Autodesk Fusion 360 part; units mm, degrees
(part 2 of 2)
  measures "d325" diameter of A232
  measures "d326" diameter of A227
  measures "d327" diameter of A198
  measures "d328" diameter of A280
  measures "d329" diameter of A253
  measures "d330" diameter of A200
  measures "d331" diameter of A269
  measures "d332" diameter of A224
  measures "d333" diameter of A233
  measures "d334" diameter of A214
  measures "d335" diameter of A265
  measures "d336" diameter of A279
  measures "d337" diameter of A204
  measures "d338" diameter of A298
  measures "d339" diameter of A210
  measures "d340" diameter of A157
  measures "d341" diameter of A205
  measures "d342" diameter of A155
  measures "d343" diameter of A225
  measures "d344" diameter of A202
  measures "d345" diameter of A241
  measures "d346" diameter of A270
  measures "d347" diameter of A262
  measures "d348" diameter of A208
  measures "d349" diameter of A301
  measures "d350" diameter of A240
  measures "d351" diameter of A197
  measures "d352" diameter of A231
  measures "d353" diameter of A264
  measures "d354" diameter of A267
  measures "d355" diameter of A213
  measures "d356" diameter of A297
  measures "d357" diameter of A164
  measures "d358" diameter of A178
  measures "d359" diameter of A194
  measures "d360" diameter of A296
  measures "d361" diameter of A180
  measures "d362" diameter of A295
  measures "d363" diameter of A182
  measures "d364" diameter of A179
  measures "d365" diameter of A192
  measures "d366" diameter of A272
  measures "d367" diameter of A277
  measures "d368" diameter of A169
  measures "d369" diameter of A154
  measures "d370" diameter of A161
  measures "d371" diameter of A259
  measures "d372" diameter of A274
  measures "d373" diameter of A184
  measures "d374" diameter of A245
  measures "d375" diameter of A167
  measures "d376" diameter of A151
  measures "d377" diameter of A168
  measures "d378" diameter of A257
  measures "d379" diameter of A256
  measures "d380" diameter of A190
  measures "d381" diameter of A299
  measures "d382" diameter of A244
  measures "d383" diameter of A189
  measures "d384" diameter of A294
  measures "d385" diameter of A282
  measures "d386" diameter of A239
  measures "d387" diameter of A234
  measures "d388" diameter of A273
  measures "d389" diameter of A271
  measures "d390" diameter of A278
  measures "d391" diameter of A230
  measures "d392" diameter of A246
  measures "d393" diameter of A228
  measures "d394" diameter of A236
  measures "d395" diameter of A242 A45.centre
  measures "d396" diameter of A207
  measures "d397" diameter of A158
  measures "d398" diameter of A186
  measures "d399" diameter of A191
  measures "d400" diameter of A199
  measures "d401" diameter of A170
  measures "d402" diameter of A219
  measures "d403" diameter of A218
  measures "d404" diameter of A211
  measures "d405" diameter of A252
  measures "d406" diameter of A258
  measures "d407" diameter of A152
  measures "d408" diameter of A254
  measures "d409" diameter of A201
  measures "d410" diameter of A222
  measures "d411" diameter of A215
  measures "d412" diameter of A261
  measures "d413" diameter of A266
  measures "d414" diameter of A217
  measures "d415" diameter of A283
  measures "d416" diameter of A196
  measures "d417" diameter of A251
  measures "d418" diameter of A185
  measures "d419" diameter of A173
  measures "d420" diameter of A159
  measures "d421" diameter of A238
  measures "d422" diameter of A209
  measures "d423" diameter of A172
  measures "d424" diameter of A177
  measures "d425" diameter of A203
  measures "d426" diameter of A220
  measures "d427" diameter of A206
  measures "d428" diameter of A249
  measures "d429" diameter of A285
  measures "d430" diameter of A174
  measures "d431" diameter of A300
  measures "d432" diameter of A226
  measures "d433" diameter of A212
  measures "d434" diameter of A235
  measures "d435" diameter of A263
  measures "d436" diameter of A291
  measures "d437" diameter of A223
  measures "d438" diameter of A255
  measures "d439" diameter of A187
  measures "d440" diameter of A176
  measures "d441" diameter of A188
  measures "d442" diameter of A243
  measures "d443" diameter of A193
  measures "d444" diameter of A195
  measures "d445" diameter of A286
  measures "d446" diameter of A288
  measures "d447" diameter of A171
  measures "d448" diameter of A153
  measures "d449" diameter of A166
  measures "d450" diameter of A290
  measures "d451" diameter of A229
  measures "d452" diameter of A181
  measures "d453" diameter of A268
  measures "d454" diameter of A160
  measures "d455" diameter of A162
  measures "d456" diameter of A156
  measures "d457" diameter of A276
  measures "d458" diameter of A237
  measures "d459" diameter of A183
  measures "d460" diameter of A250
  measures "d461" diameter of A284
  measures "d462" diameter of A275
  measures "d463" diameter of A293
  measures "d464" diameter of A248
  measures "d465" diameter of A216
  measures "d466" diameter of A260
  measures "d467" diameter of A287
  measures "d468" diameter of A292
  measures "d469" diameter of A247
  measures "d470" diameter of A289
  measures "d471" diameter of A281
  measures "d472" distance of A40.centre A62.centre
  measures "d473" diameter of A326
  measures "d474" diameter of A314
  measures "d475" diameter of A372
  measures "d476" diameter of A316
  measures "d477" diameter of A383
  measures "d478" diameter of A378
  measures "d479" diameter of A349
  measures "d480" diameter of A431
  measures "d481" diameter of A404
  measures "d482" diameter of A351
  measures "d483" diameter of A420
  measures "d484" diameter of A375
  measures "d485" diameter of A384
  measures "d486" diameter of A365
  measures "d487" diameter of A416
  measures "d488" diameter of A430
  measures "d489" diameter of A355
  measures "d490" diameter of A449
  measures "d491" diameter of A361
  measures "d492" diameter of A308
  measures "d493" diameter of A356
  measures "d494" diameter of A306
  measures "d495" diameter of A376
  measures "d496" diameter of A353
  measures "d497" diameter of A392
  measures "d498" diameter of A421
  measures "d499" diameter of A413
  measures "d500" diameter of A359
  measures "d501" diameter of A452
  measures "d502" diameter of A391
  measures "d503" diameter of A348
  measures "d504" diameter of A382
  measures "d505" diameter of A415
  measures "d506" diameter of A418
  measures "d507" diameter of A364
  measures "d508" diameter of A448
  measures "d509" diameter of A315
  measures "d510" diameter of A329
  measures "d511" diameter of A345
  measures "d512" diameter of A447
  measures "d513" diameter of A331
  measures "d514" diameter of A446
  measures "d515" diameter of A333
  measures "d516" diameter of A330
  measures "d517" diameter of A343
  measures "d518" diameter of A423 A42.centre
  measures "d519" diameter of A428
  measures "d520" diameter of A320
  measures "d521" diameter of A305
  measures "d522" diameter of A312
  measures "d523" diameter of A410
  measures "d524" diameter of A425
  measures "d525" diameter of A335
  measures "d526" diameter of A396
  measures "d527" diameter of A318
  measures "d528" diameter of A302
  measures "d529" diameter of A319
  measures "d530" diameter of A408
  measures "d531" diameter of A407
  measures "d532" diameter of A341
  measures "d533" diameter of A450
  measures "d534" diameter of A395
  measures "d535" diameter of A340
  measures "d536" diameter of A445
  measures "d537" diameter of A433
  measures "d538" diameter of A390
  measures "d539" diameter of A385
  measures "d540" diameter of A424
  measures "d541" diameter of A422
  measures "d542" diameter of A429
  measures "d543" diameter of A381
  measures "d544" diameter of A397
  measures "d545" diameter of A379
  measures "d546" diameter of A387
  measures "d547" diameter of A393
  measures "d548" diameter of A358
  measures "d549" diameter of A309
  measures "d550" diameter of A337
  measures "d551" diameter of A342
  measures "d552" diameter of A350
  measures "d553" diameter of A321
  measures "d554" diameter of A370
  measures "d555" diameter of A369
  measures "d556" diameter of A362
  measures "d557" diameter of A403
  measures "d558" diameter of A409
  measures "d559" diameter of A303
  measures "d560" diameter of A405
  measures "d561" diameter of A352
  measures "d562" diameter of A373
  measures "d563" diameter of A366
  measures "d564" diameter of A412
  measures "d565" diameter of A417
  measures "d566" diameter of A368
  measures "d567" diameter of A434
  measures "d568" diameter of A347
  measures "d569" diameter of A402
  measures "d570" diameter of A336
  measures "d571" diameter of A324
  measures "d572" diameter of A310
  measures "d573" diameter of A389
  measures "d574" diameter of A360
  measures "d575" diameter of A323
  measures "d576" diameter of A328
  measures "d577" diameter of A354
  measures "d578" diameter of A371
  measures "d579" diameter of A357
  measures "d580" diameter of A400
  measures "d581" diameter of A436
  measures "d582" diameter of A325
  measures "d583" diameter of A451
  measures "d584" diameter of A377
  measures "d585" diameter of A363
  measures "d586" diameter of A386
  measures "d587" diameter of A414
  measures "d588" diameter of A442
  measures "d589" diameter of A374
  measures "d590" diameter of A406
  measures "d591" diameter of A338
  measures "d592" diameter of A327
  measures "d593" diameter of A339
  measures "d594" diameter of A394
  measures "d595" diameter of A344
  measures "d596" diameter of A346
  measures "d597" diameter of A437
  measures "d598" diameter of A439
  measures "d599" diameter of A322
  measures "d600" diameter of A304
  measures "d601" diameter of A317
  measures "d602" diameter of A441
  measures "d603" diameter of A380
  measures "d604" diameter of A332
  measures "d605" diameter of A419
  measures "d606" diameter of A311
  measures "d607" diameter of A313
  measures "d608" diameter of A307
  measures "d609" diameter of A427
  measures "d610" diameter of A388
  measures "d611" diameter of A334
  measures "d612" diameter of A401
  measures "d613" diameter of A435
  measures "d614" diameter of A426
  measures "d615" diameter of A444
  measures "d616" diameter of A399
  measures "d617" diameter of A367
  measures "d618" diameter of A411
  measures "d619" diameter of A438
  measures "d620" diameter of A443
  measures "d621" diameter of A398
  measures "d622" diameter of A440
  measures "d623" diameter of A432
  measures "d624" distance of A331.centre A340.centre
extrude "Extrude13" cut sketch "Sketch1 (3)" against normal up to surface (193 mm away) contours A0 A3 A18 A21 A102 A139 A142 A144 A173 A175 A199 A205 A207 A209 A210 A221 | A1 A2 A19 A20 A133 A134 A137 A141 A155 A157 A158 A159 A163 A165 A170 A172 | A4 A5 A6 A9 A14 A16 A22 A23 A27 A28 A29 A30 A72 A76 A78 A79 A81 A82 A85 A89 A91 A94 A96 A97 A197 A198 A201 A202 A203 A206 A211 A212 A214 A215 A218 A219 A220 A222 A224 A225 A226 A227 A231 A232 A233 A235 A240 A241 | A7 A8 A24 A33 A103 A105 A109 A118 A152 A174 A200 A204 A208 A213 A217 A223 | A10 A17 A31 A35 A86 A101 A112 A117 A254 A255 A269 A283 A297 A298 A300 A301 | A11 A12 A25 A32 A77 A88 A92 A95 A249 A252 A261 A263 A264 A265 A270 A280 | A13 A15 A26 A34 A111 A113 A114 A116 A253 A258 A262 A266 A267 A279 A285 A291 | A36 A296 | A37 A44 A127 A129 A178 A179 A187 A193 | A38 A277 | A39 A164 | A40 A180 | A41 A43 A125 A136 A176 A192 A194 A195 | A42 A182 | A45 A46 A52 A53 A54 A55 A83 A99 A106 A108 A115 A122 A151 A153 A154 A156 A160 A161 A162 A166 A167 A168 A169 A171 | A47 A58 A75 A107 A181 A183 A184 A190 | A48 A57 A100 A104 A257 A259 A276 A290 | A49 A59 A84 A93 A229 A237 A256 A274 | A50 A295 | A51 A272 | A56 A60 A98 A119 A245 A250 A268 A299 | A61 A90 A244 A284 | A62 A189 | A63 A110 A293 A294 | A64 A80 A248 A282 | A65 A145 A216 A239 | A66 A234 | A67 A120 A273 A287 | A68 A87 A271 A292 | A69 A73 A247 A278 | A70 A121 A230 A289 | A71 A74 A246 A281 | A123 A238 | A124 A185 | A126 A243 | A128 A188 | A130 A288 | A131 A177 | A132 A275 | A135 A286 | A138 A251 | A140 A196 | A143 A228 | A146 A191 | A147 A186 | A148 A260 | A149 A242 | A150 A236 | A302 A304 A305 A307 A311 A312 A313 A317 A318 A319 A320 A322 | A303 A325 A351 A355 A359 A364 A368 A374 | A306 A308 A309 A310 A314 A316 A321 A323 | A315 | A324 A326 A350 A356 A358 A360 A361 A372 | A327 A343 A345 A346 | A328 | A329 A330 A338 A344 | A331 | A332 A334 A335 A341 | A333 | A336 | A337 | A339 | A340 | A342 | A347 | A348 A349 A352 A353 A354 A357 A362 A363 A365 A366 A369 A370 A371 A373 A375 A376 A377 A378 A382 A383 A384 A386 A391 A392 | A367 A390 | A379 | A380 A388 A407 A425 | A381 A440 | A385 | A387 | A389 | A393 | A394 | A395 A435 | A396 A401 A419 A450 | A397 A432 | A398 A429 | A399 A433 | A400 A403 A412 A414 A415 A416 A421 A431 | A402 | A404 A409 A413 A417 A418 A430 A436 A442 | A405 A406 A420 A434 A448 A449 A451 A452 | A408 A410 A427 A441 | A411 | A422 A443 | A423 | A424 A438 | A426 | A428 | A437 | A439 | A444 A445 | A446 | A447 bodies 1 in component "Box"
sketch "Sketch2 (4)" plane through (0, 0, 0) normal (0, 0, -1) x (1, 0, 0)
  circle A0 centre (-40.46, -183.46) radius 1.75
  circle A1 centre (38, -148) radius 1.75
  circle A2 centre (-40, -41) radius 1.75
  circle A3 centre (34, -92) radius 1.75
  line L0 (-50, -193) -> (80, -193)
  line L1 (80, -193) -> (80, 0)
  line L2 (80, 0) -> (-50, 0)
  line L3 (-50, 0) -> (-50, -193)
  line L4 (-19.5, -27.5) -> (49.5, -27.5)
  line L5 (49.5, -27.5) -> (49.5, -42.5)
  line L6 (49.5, -42.5) -> (-19.5, -42.5)
  line L7 (-19.5, -42.5) -> (-19.5, -27.5)
  line L8 (-19.5, -64) -> (49.5, -64)
  line L9 (49.5, -64) -> (49.5, -79)
  line L10 (49.5, -79) -> (-19.5, -79)
  line L11 (-19.5, -79) -> (-19.5, -64)
  line L12 (15, 0) -> (15, -193) construction
  line L13 (-46, -189) -> (76, -189)
  line L14 (76, -189) -> (76, -4)
  line L15 (76, -4) -> (-46, -4)
  line L16 (-46, -4) -> (-46, -189)
  circle A4 centre (15, -53.25) radius 2
  dimension "d630" = 69
  dimension "d631" = 15
  dimension "d632" = 15
  dimension "d633" = 69
  dimension "d634" = 21.5
  dimension "d635" = 34.5
  dimension "d636" = 27.5
  dimension "d642" = -4
  dimension "d665" = 4
  constraint horizontal L4
  constraint vertical L5
  constraint horizontal L6
  constraint vertical L7
  constraint horizontal L8
  constraint vertical L9
  constraint horizontal L10
  constraint vertical L11
  constraint midpoint L2 L12.start
  constraint midpoint L0 L12.end
  constraint coincident L12 A4.centre
  measures "d630" distance of L4.start L4.end
  measures "d631" distance of L4.start L6.end
  measures "d632" distance of L8.start L10.end
  measures "d633" distance of L8.start L8.end
  measures "d634" distance of L6.end L8.start
  measures "d635" distance of L4.start L12
  measures "d636" distance of L2 L4
  measures "d665" diameter of A4
extrude "Extrude19" cut sketch "Sketch2 (4)" against normal up to surface (4 mm away) contours A4 bodies 1 in component "Box"
extrude "Extrude15" add sketch "Sketch2 (4)" along normal blind 20 contours L0 L1 L2 L3 | L4 L5 L6 L7 | L8 L9 L10 L11 bodies 1 in component "Box"
sketch "Sketch3 (2)" plane through (0, 79, 0) normal (0, 1, 0) x (-1, 0, 0)
  line L0 (19.5, 0) -> (-49.5, 0)
  line L1 (-49.5, 0) -> (-49.5, -20)
  line L2 (-49.5, -20) -> (19.5, -20)
  line L3 (19.5, -20) -> (19.5, 0)
  circle A0 centre (-33.5, -13) radius 4.5
  circle A1 centre (3.5, -13) radius 4.5
  line L4 (-15, 0) -> (-15, -35) construction
  circle A2 centre (-15, -35) radius 19
  dimension "d647" = 9
  dimension "d649" = 16
  dimension "d650" = 9
  dimension "d651" = 37
  dimension "d657" = 13
  dimension "d658" = 35
  dimension "d659" = 38
  constraint midpoint L0 L4.start
  constraint perpendicular L0 L4
  constraint coincident L4.end A2.centre
  measures "d647" diameter of A0
  measures "d649" distance of L1 A0.centre
  measures "d650" diameter of A1
  measures "d651" distance of A0.centre A1.centre
  measures "d657" distance of L0 A0.centre
  measures "d658" distance of L4.start L4.end
  measures "d659" diameter of A2
extrude "Extrude18" cut sketch "Sketch3 (2)" along normal up to surface (114 mm away) and the other way up to surface (79 mm away) contours L2 A2 picked at (-15.4646, -17.6537) bodies 1 in component "Box"
extrude "Extrude16" cut sketch "Sketch3 (2)" against normal up to surface (51.5 mm away) contours A0 | A1 bodies 1 in component "Box"
extrude "Extrude11" [suppressed] in component "Box"
extrude "Extrude6" [suppressed] in component "Box"
sketch "Sketch7" plane through (0, 0, 0) normal (0, -1, 0) x (1, 0, 0) in component "Box"
  line L0 (-48.2943, 71.7234) -> (-46, 75)
  line L1 (-46, 75) -> (-50, 75)
  line L2 (-50, 75) -> (-50, 0)
  line L3 (-50, 0) -> (80, 0)
  line L4 (80, 0) -> (80, 75)
  line L5 (80, 75) -> (76, 75)
  line L6 (76, 75) -> (78.2943, 71.7234)
  line L7 (78.2943, 71.7234) -> (-48.2943, 71.7234)
  line L8 (71.52, 53.0261) -> (76.52, 53.0261)
  line L9 (76.52, 53.0261) -> (76.52, 45.0261)
  line L10 (76.52, 45.0261) -> (71.52, 53.0261)
  dimension "d86" = 8
  constraint horizontal L8
  constraint vertical L9
  measures "d86" distance of L9.end L8.end
extrude "Extrude7" [suppressed] in component "Box"
sketch "Sketch1 (4)" plane through (-46, 0, 0) normal (1, 0, 0) x (0, 1, 0) in component "Level"
  line L0 (4, 51) -> (189, 51)
  line L1 (189, 51) -> (189, 71.7234)
  line L2 (189, 71.7234) -> (4, 71.7234)
  line L3 (4, 71.7234) -> (4, 51)
component "Box" placed x (1, 0, 0) y (0, 1, 0) z (0, 0, 1) at (0, 0, 0)
component "Lid" placed x (1, 0, 0) y (0, 1, 0) z (0, 0, 1) at (0, 0, 0)
component "Level (1)" placed x (1, 0, 0) y (0, 1, 0) z (0, 0, 1) at (0, 0, 0)
equation "d1 = Length"
equation "d2 = Width"
equation "d3 = Height"
equation "d6 = Thickness"
equation "d8 = Thickness"
equation "d11 = Clearance"
equation "d12 = Clearance"
equation "Length = 193 mm"
equation "Width = 130 mm"
equation "Height = 77.5 mm"
equation "Thickness = 4 mm"
equation "Clearance = 0.3 mm"
equation "d19 = Thickness / 3"
equation "d28 = Length / 2"
equation "d66 = Switch_W"
equation "d67 = Switch_L"
equation "Switch_L = 30 mm"
equation "Switch_W = 21 mm"
equation "d96 = -Clearance"
equation "d98 = Clearance"
equation "d99 = Clearance"
equation "d630 = mount_length"
equation "d633 = mount_length"
equation "d634 = mount_width"
equation "d635 = mount_length / 2"
equation "mount_width = 21.5 mm"
equation "mount_length = 69 mm"
equation "mount_height = 20 mm"
equation "mount_screw_height = 13 mm"
equation "mount_screw_diameter = 9 mm"
equation "d643 = mount_height"
equation "mount_screw_distance = 37 mm"
equation "mount_screw_x = 16 mm"
equation "d647 = mount_screw_diameter"
equation "d649 = mount_screw_x"
equation "d650 = mount_screw_diameter"
equation "d651 = mount_screw_distance"
equation "d657 = mount_screw_height"
